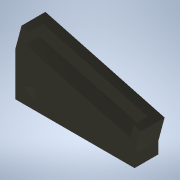
# Autodesk Inventor part: Angled Base AdapterFront
Saved by Autodesk Inventor 2020 (Build 240168000, 168)
## iProperties
Created: 2026-05-21
Part Number: Angled Base AdapterFront
Material: Generic
Document SubType Name: Modeling
Designer: sutan
Density: 1 g/cm^3
Appearance: Default
Author: sutan
Autodesk Inventor part; units mm, degrees
ref_plane "YZ Plane" through (0, 0, 0) normal (1, 0, 0) x (0, 1, 0)
ref_plane "XZ Plane" through (0, 0, 0) normal (0, 1, 0) x (-1, 0, 0)
ref_plane "XY Plane" through (0, 0, 0) normal (0, 0, 1) x (1, 0, 0)
sketch "Sketch1" plane through (0, 0, 0) normal (0, 0, 1) x (1, 0, 0)
  line L0 (-7.898, 5.9756) -> (42.102, 5.9756)
  line L1 (42.102, 5.9756) -> (42.102, -14.0244)
  line L2 (42.102, -14.0244) -> (-7.898, -14.0244)
  line L3 (-7.898, -14.0244) -> (-7.898, 5.9756)
  point P0 (0, 0)
  dimension "d0" = 50
  dimension "d1" = 20
  constraints: 8 end point, 2 parallel, 1 horizontal, 1 perpendicular
  measures "d0" distance of L1.end L2.end
  measures "d1" distance of L0.end L1.end
extrude "Extrusion1" add sketch "Sketch1" along normal blind 10
sketch "Sketch2" plane through (0, 0, 10) normal (0, 0, 1) x (1, 0, 0)
  line L0 (-7.898, 5.9756) -> (-7.898, -14.0244) projected
  line L1 (-7.898, 4.3731) -> (42.102, -9.0244)
  line L2 (42.102, -14.0244) -> (42.102, 5.9756) projected
  line L3 (-7.898, 4.3731) -> (-7.898, 5.9756)
  line L4 (42.102, 5.9756) -> (-7.898, 5.9756) projected
  line L5 (42.102, 5.9756) -> (42.102, -9.0244)
  point P0 (0, 0)
  dimension "d4" = 5
  dimension "d5" = 75
  constraints: 6 end point, 2 point on line, 1 collinear, 1 vertical
  measures "d4" distance of L2.start L1.end
  measures "d5" angle of L1 L0
extrude "Extrusion2" cut sketch "Sketch2" against normal up to surface (10 mm away)
sketch "Sketch3" plane through (-7.898, 4.3731, 10) normal (0.258819, 0.9659258, 0) x (0.9659258, -0.258819, 0)
  line L0 (53.0579, 0) -> (51.7638, 0) projected
  line L1 (0, 10) -> (4.7616, 10) projected
  line L2 (51.7638, 0) -> (0, 0)
  line L3 (0, 0) -> (0, 10)
  line L4 (0, 10) -> (51.7638, 10)
  line L5 (51.7638, 10) -> (51.7638, 0)
  point P0 (8.7608, 10)
  constraints: 8 end point, 2 parallel, 1 horizontal, 1 perpendicular
extrude "Extrusion3" add sketch "Sketch3" along normal blind 10
sketch "Sketch4" plane through (-5.3099, 14.0324, 10) normal (0.258819, 0.9659258, 0) x (0.9659258, -0.258819, 0)
  line L0 (48.632, 0) -> (3.132, 0)
  line L1 (3.132, 0) -> (3.132, 6)
  line L2 (3.132, 6) -> (48.632, 6)
  line L3 (48.632, 6) -> (48.632, 0)
  line L4 (0, 0) -> (51.7638, 0) projected
  line L5 (0, 10) -> (0, 0) projected
  line L6 (51.7638, 10) -> (0, 10) projected
  point P0 (8.7608, 10)
  point P1 (25.882, 5)
  dimension "d10" = 45.5
  dimension "d11" = 6
  dimension "d13" = 25.882
  dimension "d14" = 22.75
  dimension "d23" = 0
  constraints: 8 end point, 2 parallel, 1 horizontal, 1 perpendicular
  measures "d10" distance of L1.end L2.end
  measures "d11" distance of L0.end L1.end
  measures "d13" distance from line of L5 point (25.882, 5)
  measures "d14" distance from line of point (25.882, 5) L1
  measures "d23" distance between parallel lines of L4 L0
extrude "Extrusion4" cut sketch "Sketch4" against normal blind 5.5
sketch "Sketch5" plane through (0, 0, 10) normal (0, 0, 1) x (1, 0, 0)
  line L0 (0, -5.2088) -> (0, -10.2088)
  line L1 (0, -10.2088) -> (-4.3301, -7.7088)
  line L2 (-4.3301, -7.7088) -> (0, -5.2088)
  point P0 (0, 0)
  dimension "d17" = 5
  dimension "d18" = 5
  constraints: 6 end point, 1 vertical
  measures "d17" distance of L0.start L0.end
  measures "d18" distance of L0.end L1.end
extrude "Extrusion5" cut sketch "Sketch5" against normal blind 2.5
equation "\"d14\" = 0.5 * d10"
body "Solid1"
